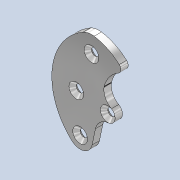
# Autodesk Inventor part: アンノーン
Saved by Autodesk Inventor 2020 (Build 240168000, 168)
## iProperties
Created: 2020-10-28
Part Number: アンノーン
Material: アルミニウム 2014-T4
Document SubType Name: Modeling
Designer: AA19065
Density: 2.8 g/cm^3
Appearance: サテン
Mass: 6.28148 g
Surface Area: 19.6323 cm^2
Volume: 2.24338 cm^3
Author: AA19065
Autodesk Inventor part; units mm, degrees
ref_plane "YZ Plane" through (0, 0, 0) normal (1, 0, 0) x (0, 1, 0)
ref_plane "XZ Plane" through (0, 0, 0) normal (0, 1, 0) x (-1, 0, 0)
ref_plane "XY Plane" through (0, 0, 0) normal (0, 0, 1) x (1, 0, 0)
sketch "スケッチ1" plane through (0, 0, 0) normal (0, 0, 1) x (1, 0, 0)
  circle A0 centre (76.2014, 18) radius 1.25
  circle A1 centre (70, 2) radius 1.5
  circle A2 centre (71.5626, -13) radius 1.25
  circle A3 centre (71.5626, -13) radius 5
  arc A4 (72.7656, 23.9999) -> (68.1729, -16.6757) centre (85.3759, 1.979) ccw
  circle A5 centre (139.7986, 18) radius 1.25
  circle A6 centre (139.7986, 18) radius 6.914
  arc A7 (147.8271, -16.6757) -> (143.2344, 23.9999) centre (130.6241, 1.979) ccw
  circle A8 centre (146, 2) radius 1.5
  circle A9 centre (144.4374, -13) radius 5
  circle A10 centre (144.4374, -13) radius 1.25
  circle A11 centre (76.2014, 18) radius 6.914
  line L0 (82.9641, 16.5612) -> (76.4531, -14.0405)
  line L1 (133.0359, 16.5612) -> (139.5469, -14.0405)
  arc A12 (87.1691, 16.7068) -> (81.2992, 8.7363) centre (93.0365, 6.239) ccw
  arc A13 (87.1691, 16.7068) -> (87.5297, 19.9375) centre (86.1912, 18.4514) ccw
  arc A14 (87.5297, 19.9375) -> (77.288, 24.8281) centre (74.1449, 5.0766) ccw
  line L2 (108, 72.8318) -> (108, -27.6373) construction
  arc A15 (134.7008, 8.7363) -> (128.8309, 16.7068) centre (122.9635, 6.239) ccw
  arc A16 (138.712, 24.8281) -> (128.4703, 19.9375) centre (141.8551, 5.0766) ccw
  arc A17 (128.4703, 19.9375) -> (128.8309, 16.7068) centre (129.8088, 18.4514) ccw
  circle A18 centre (82.8568, 0.0761) radius 1.5
  circle A19 centre (133.1432, 0.0761) radius 1.75
  circle A20 centre (82.8568, 0.0761) radius 3
  arc A21 (81.3922, 9.1736) -> (84.3249, 2.6924) centre (87.2609, 7.9249) ccw
  arc A22 (83.1326, -2.9112) -> (77.8155, -7.6372) centre (83.6841, -8.8858) ccw
  arc A23 (131.6751, 2.6924) -> (134.6078, 9.1736) centre (128.7391, 7.9249) ccw
  circle A24 centre (133.1432, 0.0761) radius 3
  arc A25 (138.1845, -7.6372) -> (132.8674, -2.9112) centre (132.3159, -8.8858) ccw
  circle A26 centre (76.2014, 18) radius 1.5
  circle A27 centre (71.5626, -13) radius 1.5
  point P0 (0, 0)
  point P1 (0, 0)
  point P2 (81.3565, 8.9919)
  dimension "d0" = 8
  dimension "d1" = 2
  dimension "d2" = 12
  dimension "d3" = 20
  dimension "d4" = 10
  dimension "d5" = 6
  dimension "d6" = 6
  dimension "d7" = 6
  dimension "d10" = 2.5
  dimension "d11" = 3
  dimension "d12" = 3
  dimension "d13" = 3
  constraints: 35 point on circle, 28 centre point, 14 symmetric about line, 12 tangent, 6 end point, 3 coincident, 3 point on line, 14 other
  measures "d0" distance of A12.end L0.start
  measures "d1" radius of A13
  measures "d2" radius of A12
  measures "d3" radius of A14
  measures "d4" distance of A0.centre A13.centre
  measures "d5" diameter of A20
  measures "d6" radius of A21
  measures "d7" radius of A22
  measures "d10" diameter of A0
  measures "d11" diameter of A26
  measures "d12" diameter of A27
  measures "d13" diameter of A18
extrude "押し出し1" add sketch "スケッチ1" along normal blind 3 contours A3 | A3 A4 A11 L0 | A11 | L0 A12 A21 A20 A22 | A14 A13 A12 A21 L0 A11 | A20
equation "\"d7\" = d6"
